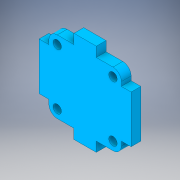
# Autodesk Inventor part: HGLRC Micro 13A 4in1 BLHeli_S
Saved by Autodesk Inventor 2018 (Build 220112000, 112)
## iProperties
Created: 2018-01-27
Part Number: HGLRC Micro 13A 4in1 BLHeli_S
Material: Všeobecné
Document SubType Name: Modeling
Designer: Kuba
Density: 1 g/cm^3
Appearance: Výchozí
Author: Kuba
Autodesk Inventor part; units mm, degrees
ref_plane "YZ Plane" through (0, 0, 0) normal (1, 0, 0) x (0, 1, 0)
ref_plane "XZ Plane" through (0, 0, 0) normal (0, 1, 0) x (-1, 0, 0)
ref_plane "XY Plane" through (0, 0, 0) normal (0, 0, 1) x (1, 0, 0)
sketch "Sketch2" plane through (0, 0, 0) normal (0, 1, 0) x (-1, 0, 0)
  line L0 (10, -13) -> (-10, -13)
  line L1 (-13, -10) -> (-13, 10)
  line L2 (-10, 13) -> (10, 13)
  line L3 (13, 10) -> (13, -10)
  line L4 (13, -13) -> (-13, 13) construction
  line L5 (-13, -13) -> (13, 13) construction
  circle A0 centre (10, 10) radius 1.5
  circle A1 centre (-10, 10) radius 1.5
  circle A2 centre (-10, -10) radius 1.5
  circle A3 centre (10, -10) radius 1.5
  arc A4 (13, 10) -> (10, 13) centre (10, 10) ccw
  arc A5 (-10, 13) -> (-13, 10) centre (-10, 10) ccw
  arc A6 (-13, -10) -> (-10, -13) centre (-10, -10) ccw
  arc A7 (10, -13) -> (13, -10) centre (10, -10) ccw
  line L6 (13, 8.5) -> (16.5, 8.5)
  line L7 (16.5, 8.5) -> (16.5, -8.5)
  line L8 (16.5, -8.5) -> (13, -8.5)
  line L9 (13, -8.5) -> (13, 8.5)
  line L10 (0, 0) -> (6.0959, 0)
  line L11 (0, 0) -> (0, 5.3302)
  line L12 (-13, 8.5) -> (-16.5, 8.5)
  line L13 (-16.5, 8.5) -> (-16.5, -8.5)
  line L14 (-16.5, -8.5) -> (-13, -8.5)
  line L15 (-13, -8.5) -> (-13, 8.5)
  line L16 (4, 13) -> (-4, 13)
  line L17 (-4, 13) -> (-4, 16.5)
  line L18 (-4, 16.5) -> (4, 16.5)
  line L19 (4, 16.5) -> (4, 13)
  line L20 (4, -13) -> (-4, -13)
  line L21 (-4, -13) -> (-4, -16.5)
  line L22 (-4, -16.5) -> (4, -16.5)
  line L23 (4, -16.5) -> (4, -13)
  dimension "d10" = 26
  dimension "d11" = 26
  dimension "d12" = 3
  dimension "d13" = 3
  dimension "d14" = 3
  dimension "d15" = 3
  dimension "d16" = 20
  dimension "d17" = 3
  dimension "d18" = 3.5
  dimension "d19" = 17
  dimension "d20" = 8
  dimension "d21" = 3.5
  constraints: 48 end point, 14 point on line, 8 centre point, 8 point on circle, 8 symmetric about line, 8 tangent, 6 parallel, 4 horizontal, 3 equal radius, 3 perpendicular, 2 horizontal alignment, 2 midpoint, 2 vertical alignment, 1 vertical, 2 other
  measures "d10" distance of L4.end L5.end
  measures "d11" distance of L5.start L4.end
  measures "d12" diameter of A0
  measures "d13" diameter of A1
  measures "d14" diameter of A2
  measures "d15" diameter of A3
  measures "d16" distance of A1.centre A0.centre
  measures "d17" radius of A4
  measures "d18" distance of L7.end L8.end
  measures "d19" distance of L6.end L7.end
  measures "d20" distance of L17.end L18.end
  measures "d21" distance of L16.end L17.end
extrude "Extrusion2" add sketch "Sketch2" along normal blind 3.5
body "Solid2"
